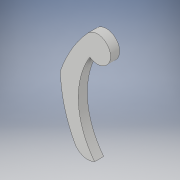
# Autodesk Inventor part: BHENCHOD FINGER
Saved by Autodesk Inventor 2017 (Build 210142000, 142)
## iProperties
Created: 2017-11-30
Part Number: BHENCHOD FINGER
Material: Generic
Document SubType Name: Modeling
Designer: Sam
Density: 1 g/cm^3
Appearance: Default
Author: Sam
Autodesk Inventor part; units mm, degrees
ref_plane "YZ Plane" through (0, 0, 0) normal (1, 0, 0) x (0, 1, 0)
ref_plane "XZ Plane" through (0, 0, 0) normal (0, 1, 0) x (-1, 0, 0)
ref_plane "XY Plane" through (0, 0, 0) normal (0, 0, 1) x (1, 0, 0)
sketch "Sketch1" plane through (0, 0, 0) normal (0, 0, 1) x (1, 0, 0)
  arc A0 (-46.1263, 10.632) -> (-62.6331, -17.4708) centre (15.0732, -44.2142) ccw projected
  arc A1 (-62.6331, -17.4708) -> (-54.2395, -22.9066) centre (-57.7619, -19.1473) ccw projected
  arc A2 (-33.338, 11.3144) -> (-54.2395, -22.9066) centre (22.5624, -46.3221) ccw projected
  arc A3 (-33.338, 11.3144) -> (-46.1263, 10.632) centre (-39.3918, 4.5967) ccw construction
  arc A4 (-62.8989, -19.5348) -> (-54.0515, -50.903) centre (19.0478, -13.3535) ccw projected
  arc A5 (-54.0515, -50.903) -> (-41.8534, -54.8035) centre (-46.0076, -46.7711) ccw projected
  arc A6 (-53.4019, -16.4032) -> (-41.8534, -54.8035) centre (26.8267, -13.212) ccw projected
  arc A7 (-53.4019, -16.4032) -> (-62.8989, -19.5348) centre (-57.7619, -19.1473) ccw projected
  arc A8 (-29.559, -59.3436) -> (2.6139, -54.1332) centre (-26.3493, 22.7733) ccw projected
  arc A9 (2.6139, -54.1332) -> (1.4472, -44.2015) centre (0.7983, -49.3121) ccw projected
  arc A10 (-38.241, -49.9292) -> (1.4472, -44.2015) centre (-29.5023, 29.8859) ccw projected
  arc A11 (-38.241, -49.9292) -> (-29.559, -59.3436) centre (-29.2058, -50.3074) ccw projected
  arc A12 (4.4376, -52.9584) -> (22.4821, -25.8173) centre (-53.6163, 5.2072) ccw projected
  arc A13 (22.4821, -25.8173) -> (17.499, -14.02) centre (14.1082, -22.4033) ccw projected
  arc A14 (-4.1234, -47.7902) -> (17.499, -14.02) centre (-58.7892, 11.0185) ccw projected
  arc A15 (-4.1234, -47.7902) -> (4.4376, -52.9584) centre (0.7983, -49.3121) ccw projected
  arc A16 (-44.7504, -1.2652) -> (-41.8534, -54.8035) centre (-4.8947, -25.9562) ccw
  arc A17 (-46.1263, 10.632) -> (-62.6331, -17.4708) centre (15.0732, -44.2142) ccw
  arc A18 (-62.6331, -17.4708) -> (-54.0515, -50.903) centre (13.2398, -15.8127) ccw
  arc A19 (-54.0515, -50.903) -> (-41.8534, -54.8035) centre (-46.0076, -46.7711) ccw
  circle A20 centre (-40.1686, 5.2928) radius 8
  arc A21 (-44.7504, -1.2652) -> (-41.8534, -54.8035) centre (-4.8947, -25.9562) ccw
  arc A22 (-46.1263, 10.632) -> (-44.7504, -1.2652) centre (-40.1686, 5.2928) ccw
  point P0 (0, 0)
  dimension "d4" = 16
  constraints: 12 point on circle, 6 centre point, 2 concentric, 2 tangent, 6 other
extrude "Extrusion3" add sketch "Sketch1" along normal blind 5.5 contours A20 A16 A2 A6 A7 A0 | A20 A2 | A7 A6 A2 A1 A18 | A20 A2 | A1 A2 A6 A16 A5 A4 A18 | A16 A6 A2 | A4 A18
body "Solid3"
